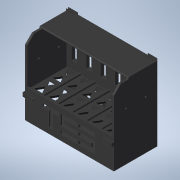
# Autodesk Inventor part: controllbox_1_copy
Saved by Autodesk Inventor 2020 (Build 240168000, 168)
## iProperties
Created: 2020-05-26
Part Number: controllbox_1_copy
Material: Generic
Document SubType Name: Modeling
Designer: Gebruiker
Density: 1 g/cm^3
Appearance: Default
Author: Gebruiker
Autodesk Inventor part; units mm, degrees
ref_plane "YZ Plane" through (0, 0, 0) normal (1, 0, 0) x (0, 1, 0)
ref_plane "XZ Plane" through (0, 0, 0) normal (0, 1, 0) x (-1, 0, 0)
ref_plane "XY Plane" through (0, 0, 0) normal (0, 0, 1) x (1, 0, 0)
sketch "Sketch1" plane through (0, 0, 0) normal (0, 0, 1) x (1, 0, 0)
  line L0 (-122.5, 65) -> (122.5, 65)
  line L1 (122.5, 65) -> (122.5, -65)
  line L2 (122.5, -65) -> (-122.5, -65)
  line L3 (-122.5, -65) -> (-122.5, 65)
  line L4 (-122.5, 65) -> (122.5, -65) construction
  line L5 (122.5, 65) -> (-122.5, -65) construction
  line L6 (-109, -65) -> (-109, 65) construction
  line L7 (-122.5, -56) -> (122.5, -56) construction
  circle A0 centre (-109, -56) radius 2
  circle A1 centre (-109, 42) radius 2
  line L8 (-109, 42) -> (122.5, 42) construction
  circle A2 centre (-69, -56) radius 2
  circle A3 centre (-29, -56) radius 2
  circle A4 centre (11, -56) radius 2
  circle A5 centre (51, -56) radius 2
  circle A6 centre (91, -56) radius 2
  line L9 (0, 65) -> (0, -65) construction
  circle A7 centre (-69, 42) radius 2
  circle A8 centre (-29, 42) radius 2
  circle A9 centre (11, 42) radius 2
  circle A10 centre (51, 42) radius 2
  circle A11 centre (91, 42) radius 2
  line L10 (-29, 42) -> (-29, -56) construction
  line L11 (-97, 65) -> (-97, -65) construction
  line L12 (-122.5, -1) -> (122.5, -1) construction
  line L13 (-104.5, 36.5) -> (-89.5, 36.5)
  line L14 (-89.5, 36.5) -> (-89.5, -38.5)
  line L15 (-89.5, -38.5) -> (-104.5, -38.5)
  line L16 (-104.5, -38.5) -> (-104.5, 36.5)
  line L17 (-104.5, 36.5) -> (-89.5, -38.5) construction
  line L18 (-89.5, 36.5) -> (-104.5, -38.5) construction
  line L19 (-64.5, 36.5) -> (-49.5, 36.5)
  line L20 (-49.5, 36.5) -> (-49.5, -38.5)
  line L21 (-64.5, -38.5) -> (-64.5, 36.5)
  line L22 (-49.5, -38.5) -> (-64.5, -38.5)
  line L23 (-24.5, 36.5) -> (-9.5, 36.5)
  line L24 (-9.5, 36.5) -> (-9.5, -38.5)
  line L25 (-24.5, -38.5) -> (-24.5, 36.5)
  line L26 (-9.5, -38.5) -> (-24.5, -38.5)
  line L27 (15.5, 36.5) -> (30.5, 36.5)
  line L28 (30.5, 36.5) -> (30.5, -38.5)
  line L29 (15.5, -38.5) -> (15.5, 36.5)
  line L30 (30.5, -38.5) -> (15.5, -38.5)
  line L31 (55.5, 36.5) -> (70.5, 36.5)
  line L32 (70.5, 36.5) -> (70.5, -38.5)
  line L33 (55.5, -38.5) -> (55.5, 36.5)
  line L34 (70.5, -38.5) -> (55.5, -38.5)
  line L35 (95.5, 36.5) -> (110.5, 36.5)
  line L36 (110.5, 36.5) -> (110.5, -38.5)
  line L37 (95.5, -38.5) -> (95.5, 36.5)
  line L38 (110.5, -38.5) -> (95.5, -38.5)
  line L39 (-105, 60.0133) -> (105, 60.0133)
  line L40 (105, 60.0133) -> (105, 50.0133)
  line L41 (105, 50.0133) -> (-105, 50.0133)
  line L42 (-105, 50.0133) -> (-105, 60.0133)
  line L43 (-105, 60.0133) -> (105, 50.0133) construction
  line L44 (105, 60.0133) -> (-105, 50.0133) construction
  point P0 (0, 0)
  point P1 (-97, -1)
  point P2 (0, 55.0133)
  dimension "d0" = 245
  dimension "d1" = 130
  dimension "d20" = 13.5
  dimension "d21" = 9
  dimension "d22" = 4
  dimension "d23" = 4
  dimension "d24" = 98
  dimension "d27" = 40
  dimension "d32" = 31.5
  dimension "d35" = 40
  dimension "d43" = 12
  dimension "d44" = 43
  dimension "d45" = 15
  dimension "d46" = 75
  dimension "d49" = 40
  dimension "d56" = 210
  dimension "d57" = 10
  dimension "d61" = 9
  constraints: 90 end point, 15 point on line, 12 centre point, 8 midpoint, 8 perpendicular, 6 horizontal, 6 parallel, 60 other
  measures "d0" distance of L1.end L2.end
  measures "d1" distance of L0.end L1.end
  measures "d20" distance between parallel lines of L6 L3
  measures "d21" distance between parallel lines of L7 L2
  measures "d22" diameter of A0
  measures "d23" diameter of A1
  measures "d24" distance of A0.centre L8.start
  measures "d27" distance of A0.centre A2.centre
  measures "d32" distance from line of L1 A6.centre
  measures "d35" distance of L8.start A7.centre
  measures "d43" distance from line of L11 L8.start
  measures "d44" distance from line of L12 L8.start
  measures "d45" distance of L14.end L15.end
  measures "d46" distance of L13.end L14.end
  measures "d49" distance of L13.start L19.start
  measures "d56" distance of L40.end L41.end
  measures "d57" distance of L39.end L40.end
  measures "d61" distance of L6.start A0.centre
extrude "Extrusion1" add sketch "Sketch1" against normal blind 10 contours L0 L1 L2 L3 | A0 | A1 | A2 | A3 | A4 | A5 | A6 | A7 | A8 | A9 | A10 | A11 | L13 L14 L15 L16 | L19 L20 L22 L21 | L23 L24 L26 L25 | L27 L28 L30 L29 | L31 L32 L34 L33 | L35 L36 L38 L37 | L39 L40 L41 L42
sketch "Sketch2" plane through (122.5, -65, 0) normal (1, 0, 0) x (0, 0, -1)
  line L0 (0, 0) -> (0, 130) projected
  line L1 (0, 0) -> (-110, 0)
  line L2 (-110, 0) -> (-110, 10)
  line L3 (-110, 10) -> (0, 10)
  line L4 (0, 10) -> (0, 0)
  point P0 (0, 65)
  dimension "d4" = 110
  dimension "d5" = 10
  constraints: 8 end point, 2 parallel, 1 horizontal, 1 perpendicular
  measures "d4" distance of L2.end L3.end
  measures "d5" distance of L1.end L2.end
extrude "Extrusion2" add sketch "Sketch2" against normal blind 245
sketch "Sketch3" plane through (122.5, -55, 110) normal (0, 1, 0) x (1, 0, 0)
  line L0 (0, 110) -> (-245, 110) projected
  line L1 (-240, 110) -> (-205, 110)
  line L2 (-205, 110) -> (-205, 5)
  line L3 (-205, 5) -> (-240, 5)
  line L4 (-240, 5) -> (-240, 110)
  line L5 (-245, 0) -> (-245, 110) projected
  line L6 (-245, 120) -> (-245, 0) projected
  line L7 (-245, 60) -> (0, 60) construction
  line L8 (0, 0) -> (0, 120) projected
  line L9 (-200, 110) -> (-165, 110)
  line L10 (-165, 110) -> (-165, 5)
  line L11 (-165, 5) -> (-200, 5)
  line L12 (-200, 5) -> (-200, 110)
  line L13 (-160, 110) -> (-125, 110)
  line L14 (-125, 110) -> (-125, 5)
  line L15 (-125, 5) -> (-160, 5)
  line L16 (-160, 5) -> (-160, 110)
  line L17 (-122.5, 110) -> (-122.5, 0) construction
  line L18 (0, 0) -> (-245, 0) construction
  line L19 (-40, 110) -> (-40, 5)
  line L20 (-40, 5) -> (-5, 5)
  line L21 (-5, 5) -> (-5, 110)
  line L22 (-80, 110) -> (-80, 5)
  line L23 (-80, 5) -> (-45, 5)
  line L24 (-45, 5) -> (-45, 110)
  line L25 (-120, 110) -> (-120, 5)
  line L26 (-120, 5) -> (-85, 5)
  line L27 (-85, 5) -> (-85, 110)
  line L28 (-234.4661, 12.7611) -> (-210.5339, 12.7611)
  line L29 (-210.5339, 12.7611) -> (-222.5, 33.6484)
  line L30 (-222.5, 33.6484) -> (-234.4661, 12.7611)
  line L31 (-222.5, 37.4721) -> (-234.4661, 56.2033)
  line L32 (-234.4661, 56.2033) -> (-210.5339, 56.2033)
  line L33 (-210.5339, 56.2033) -> (-222.5, 37.4721)
  line L34 (-210.5339, 107.2389) -> (-222.5, 86.3516)
  line L35 (-222.5, 86.3516) -> (-234.4661, 107.2389)
  line L36 (-222.5, 82.5279) -> (-234.4661, 63.7967)
  line L37 (-234.4661, 63.7967) -> (-210.5339, 63.7967)
  line L38 (-210.5339, 63.7967) -> (-222.5, 82.5279)
  line L39 (-234.4661, 107.2389) -> (-210.5339, 107.2389)
  line L40 (-205, 110) -> (-200, 110) construction
  line L41 (-200, 110) -> (-200, 5) construction
  line L42 (-200, 5) -> (-205, 5) construction
  line L43 (-205, 5) -> (-205, 110) construction
  line L44 (-202.5, 110) -> (-202.5, 5) construction
  line L45 (-170.5339, 12.7611) -> (-194.4661, 12.7611)
  line L46 (-194.4661, 12.7611) -> (-182.5, 33.6484)
  line L47 (-182.5, 33.6484) -> (-170.5339, 12.7611)
  line L48 (-182.5, 37.4721) -> (-170.5339, 56.2033)
  line L49 (-170.5339, 56.2033) -> (-194.4661, 56.2033)
  line L50 (-194.4661, 56.2033) -> (-182.5, 37.4721)
  line L51 (-194.4661, 63.7967) -> (-182.5, 82.5279)
  line L52 (-170.5339, 63.7967) -> (-194.4661, 63.7967)
  line L53 (-182.5, 82.5279) -> (-170.5339, 63.7967)
  line L54 (-182.5, 86.3516) -> (-170.5339, 107.2389)
  line L55 (-194.4661, 107.2389) -> (-182.5, 86.3516)
  line L56 (-170.5339, 107.2389) -> (-194.4661, 107.2389)
  line L57 (-165, 110) -> (-160, 110) construction
  line L58 (-160, 110) -> (-160, 5) construction
  line L59 (-160, 5) -> (-165, 5) construction
  line L60 (-165, 5) -> (-165, 110) construction
  line L61 (-162.5, 110) -> (-162.5, 5) construction
  line L62 (-130.5339, 12.7611) -> (-142.5, 33.6484)
  line L63 (-142.5, 33.6484) -> (-154.4661, 12.7611)
  line L64 (-154.4661, 12.7611) -> (-130.5339, 12.7611)
  line L65 (-142.5, 37.4721) -> (-154.4661, 56.2033)
  line L66 (-130.5339, 56.2033) -> (-142.5, 37.4721)
  line L67 (-154.4661, 56.2033) -> (-130.5339, 56.2033)
  line L68 (-154.4661, 63.7967) -> (-130.5339, 63.7967)
  line L69 (-130.5339, 63.7967) -> (-142.5, 82.5279)
  line L70 (-142.5, 82.5279) -> (-154.4661, 63.7967)
  line L71 (-142.5, 86.3516) -> (-154.4661, 107.2389)
  line L72 (-130.5339, 107.2389) -> (-142.5, 86.3516)
  line L73 (-154.4661, 107.2389) -> (-130.5339, 107.2389)
  line L74 (-10.5339, 12.7611) -> (-34.4661, 12.7611)
  line L75 (-22.5, 33.6484) -> (-10.5339, 12.7611)
  line L76 (-22.5, 37.4721) -> (-10.5339, 56.2033)
  line L77 (-10.5339, 56.2033) -> (-34.4661, 56.2033)
  line L78 (-34.4661, 56.2033) -> (-22.5, 37.4721)
  line L79 (-34.4661, 63.7967) -> (-22.5, 82.5279)
  line L80 (-10.5339, 63.7967) -> (-34.4661, 63.7967)
  line L81 (-22.5, 82.5279) -> (-10.5339, 63.7967)
  line L82 (-22.5, 86.3516) -> (-10.5339, 107.2389)
  line L83 (-34.4661, 107.2389) -> (-22.5, 86.3516)
  line L84 (-10.5339, 107.2389) -> (-34.4661, 107.2389)
  line L85 (-50.5339, 12.7611) -> (-62.5, 33.6484)
  line L86 (-74.4661, 12.7611) -> (-50.5339, 12.7611)
  line L87 (-62.5, 37.4721) -> (-74.4661, 56.2033)
  line L88 (-50.5339, 56.2033) -> (-62.5, 37.4721)
  line L89 (-74.4661, 56.2033) -> (-50.5339, 56.2033)
  line L90 (-74.4661, 63.7967) -> (-50.5339, 63.7967)
  line L91 (-50.5339, 63.7967) -> (-62.5, 82.5279)
  line L92 (-62.5, 82.5279) -> (-74.4661, 63.7967)
  line L93 (-62.5, 86.3516) -> (-74.4661, 107.2389)
  line L94 (-50.5339, 107.2389) -> (-62.5, 86.3516)
  line L95 (-74.4661, 107.2389) -> (-50.5339, 107.2389)
  line L96 (-102.5, 33.6484) -> (-90.5339, 12.7611)
  line L97 (-90.5339, 12.7611) -> (-114.4661, 12.7611)
  line L98 (-114.4661, 12.7611) -> (-102.5, 33.6484)
  line L99 (-114.4661, 56.2033) -> (-102.5, 37.4721)
  line L100 (-102.5, 37.4721) -> (-90.5339, 56.2033)
  line L101 (-90.5339, 56.2033) -> (-114.4661, 56.2033)
  line L102 (-90.5339, 63.7967) -> (-114.4661, 63.7967)
  line L103 (-102.5, 82.5279) -> (-90.5339, 63.7967)
  line L104 (-114.4661, 63.7967) -> (-102.5, 82.5279)
  line L105 (-114.4661, 107.2389) -> (-102.5, 86.3516)
  line L106 (-102.5, 86.3516) -> (-90.5339, 107.2389)
  line L107 (-90.5339, 107.2389) -> (-114.4661, 107.2389)
  line L108 (-74.4661, 12.7611) -> (-62.5, 33.6484)
  line L109 (-34.4661, 12.7611) -> (-22.5, 33.6484)
  dimension "d8" = 35
  dimension "d9" = 105
  dimension "d10" = 5
  dimension "d11" = 35
  dimension "d12" = 35
  dimension "d13" = 105
  dimension "d14" = 5
  dimension "d15" = 5
  constraints: 210 end point, 78 symmetric about line, 10 parallel, 8 horizontal, 7 midpoint, 5 perpendicular, 3 equal length, 3 point on line
  measures "d8" distance of L2.end L3.end
  measures "d9" distance of L1.end L2.end
  measures "d10" distance between parallel lines of L4 L5
  measures "d11" distance of L10.end L11.end
  measures "d12" distance of L14.end L15.end
  measures "d13" distance of L13.end L14.end
  measures "d14" distance between parallel lines of L12 L2
  measures "d15" distance between parallel lines of L16 L10
extrude "Extrusion3" cut sketch "Sketch3" against normal blind 5 contours L21 L20 L19 L0 | L2 L3 L4 L0 | L10 L11 L12 L0 | L14 L15 L16 L0 | L27 L26 L25 L0 | L24 L23 L22 L0 | L30 L29 L28 | L31 L32 L33 | L34 L35 L39 | L38 L37 L36 | L45 L46 L47 | L50 L49 L48 | L51 L53 L52 | L55 L56 L54 | L64 L63 L62 | L65 L67 L66 | L70 L69 L68 | L71 L73 L72 | L74 L109 L75 | L78 L77 L76 | L79 L81 L80 | L83 L84 L82 | L86 L108 L85 | L87 L89 L88 | L92 L91 L90 | L93 L95 L94 | L96 L97 L98 | L101 L100 L99 | L102 L104 L103 | L107 L106 L105
extrude "Extrusion4" cut sketch "Sketch3" against normal blind 10 contours L30 L29 L28 | L31 L32 L33 | L34 L35 L39 | L38 L37 L36 | L45 L46 L47 | L50 L49 L48 | L51 L53 L52 | L55 L56 L54 | L64 L63 L62 | L65 L67 L66 | L70 L69 L68 | L71 L73 L72 | L74 L109 L75 | L78 L77 L76 | L79 L81 L80 | L83 L84 L82 | L86 L108 L85 | L87 L89 L88 | L92 L91 L90 | L93 L95 L94 | L96 L97 L98 | L101 L100 L99 | L102 L104 L103 | L107 L106 L105
extrude "Extrusion5" cut sketch "Sketch1" against normal blind 10 contours A0 | A1 | A2 | A3 | A4 | A5 | A6 | A7 | A8 | A9 | A10 | A11
extrude "Extrusion6" cut sketch "Sketch1" against normal blind 10 contours L13 L14 L15 L16 | L19 L20 L22 L21 | L23 L24 L26 L25 | L27 L28 L30 L29 | L31 L32 L34 L33 | L35 L36 L38 L37
extrude "Extrusion7" cut sketch "Sketch1" against normal blind 10 contours L39 L40 L41 L42
fillet "Fillet1" radius 2 4 edges at (-105, 50.0133, -5) (-105, 60.0133, -5) (105, 50.0133, -5) (105, 60.0133, -5)
sketch "Sketch4" plane through (122.5, -65, 110) normal (0, 0, 1) x (1, 0, 0)
  line L0 (0, 10) -> (-245, 10) projected
  line L1 (-245, 10) -> (-240, 10)
  line L2 (-240, 10) -> (-240, 130)
  line L3 (-240, 130) -> (-245, 130)
  line L4 (-245, 130) -> (-245, 10)
  line L5 (0, 130) -> (-245, 130) projected
  line L6 (0, 10) -> (-5, 10)
  line L7 (-5, 10) -> (-5, 130)
  line L8 (-5, 130) -> (0, 130)
  line L9 (0, 130) -> (0, 10)
  line L10 (0, 120) -> (0, 125)
  point P0 (-122.5, 65)
  point P1 (-245, 125)
  dimension "d62" = 5
  dimension "d63" = 120
  dimension "d64" = 0
  dimension "d66" = 120
  dimension "d69" = 5
  constraints: 18 end point, 4 parallel, 2 horizontal, 2 perpendicular
  measures "d62" distance of L3.end L2.end
  measures "d63" distance of L2.end L1.end
  measures "d64" distance between parallel lines of L5 L3
  measures "d66" distance of L6.end L7.end
  measures "d69" distance of L10.end L10.start
extrude "Extrusion8" add sketch "Sketch4" against normal blind 110 contours L0 L7 L5 L9 | L0 L4 L3 L2
sketch "Sketch5" plane through (122.5, -65, -10) normal (1, 0, 0) x (0, 0, -1)
  line L0 (0, 0) -> (0, 130) projected
  line L1 (0, 130) -> (-80, 130)
  line L2 (-80, 130) -> (-80, 135)
  line L3 (-80, 135) -> (0, 135)
  line L4 (0, 135) -> (0, 130)
  point P0 (-10, 65)
  dimension "d70" = 80
  dimension "d71" = 5
  constraints: 8 end point, 2 parallel, 1 horizontal, 1 perpendicular
  measures "d70" distance of L2.end L3.end
  measures "d71" distance of L1.end L2.end
extrude "Extrusion9" add sketch "Sketch5" against normal blind 245
fillet "Fillet2" radius 2 4 edges at (120, 65, 70) (0, 70, 70) (-120, 65, 70) (0, 65, 70)
sketch "Sketch11" plane through (-122.5, -65, -10) normal (0, -1, 0) x (1, 0, 0)
  line L0 (0, 0) -> (0, 120) projected
  line L1 (245, 120) -> (245, 0) projected
  line L2 (0, 0) -> (245, 0)
  line L3 (245, 0) -> (245, 5)
  line L4 (245, 5) -> (0, 5)
  line L5 (0, 5) -> (0, 0)
  line L6 (240, 120) -> (240, 115) projected
  line L7 (245, 0) -> (240, 0)
  line L8 (240, 0) -> (240, 120)
  line L9 (240, 120) -> (245, 120)
  line L10 (245, 120) -> (245, 0)
  line L11 (245, 120) -> (0, 120) projected
  line L12 (245, 120) -> (0, 120)
  line L13 (0, 120) -> (0, 115)
  line L14 (0, 115) -> (245, 115)
  line L15 (245, 115) -> (245, 120)
  point P0 (122.5, 10)
  point P1 (240, 5)
  dimension "d103" = 5
  constraints: 24 end point, 6 parallel, 3 horizontal, 3 perpendicular, 2 point on line
  measures "d103" distance of L3.end L2.end
extrude "Extrusion13" add sketch "Sketch11" along normal blind 65 contours L0 L4 L8 L2 | L8 L4 L1 L2 | L0 L11 L6 L14 | L8 L14 L1 L4 | L6 L9 L1 L14
sketch "Sketch12" plane through (122.5, 70, 68) normal (1, 0, 0) x (0, 0, -1)
  line L0 (78, -200) -> (-42, -200) projected
  line L1 (78, -200) -> (-42, -200)
  line L2 (-42, -200) -> (-42, -205)
  line L3 (-42, -205) -> (78, -205)
  line L4 (78, -205) -> (78, -200)
  point P0 (68, -70)
  dimension "d106" = 5
  constraints: 8 end point, 2 parallel, 1 horizontal, 1 perpendicular
  measures "d106" distance of L2.end L1.end
extrude "Extrusion14" add sketch "Sketch12" against normal blind 245
sketch "Sketch13" plane through (117.5, -55, 110) normal (0, 0, 1) x (1, 0, 0)
  line L0 (-240, 125) -> (-240, -80) construction
  line L1 (5, 120) -> (5, -80) construction
  line L2 (5, -80) -> (-240, -80) construction
  line L3 (5, -0.0002) -> (-240, -80) construction
  line L4 (-240, -40.0001) -> (5, -40.0001) construction
  line L5 (-192.5, -15.0001) -> (-42.5, -15.0001)
  line L6 (-42.5, -15.0001) -> (-42.5, -65.0001)
  line L7 (-42.5, -65.0001) -> (-192.5, -65.0001)
  line L8 (-192.5, -65.0001) -> (-192.5, -15.0001)
  line L9 (-42.5, -15.0001) -> (-192.5, -65.0001) construction
  line L10 (-192.5, -15.0001) -> (-147.5, -15.0001)
  line L11 (-147.5, -15.0001) -> (-147.5, -25.0001)
  line L12 (-147.5, -25.0001) -> (-192.5, -25.0001)
  line L13 (-192.5, -25.0001) -> (-192.5, -15.0001)
  line L14 (-175, -15.0001) -> (-165, -15.0001)
  line L15 (-165, -15.0001) -> (-165, -65.0001)
  line L16 (-165, -65.0001) -> (-175, -65.0001)
  line L17 (-175, -65.0001) -> (-175, -15.0001)
  line L18 (-175, -15.0001) -> (-165, -65.0001) construction
  line L19 (-165, -15.0001) -> (-175, -65.0001) construction
  line L20 (-97.5, -15.0001) -> (-142.5, -15.0001)
  line L21 (-142.5, -15.0001) -> (-142.5, -25.0001)
  line L22 (-142.5, -25.0001) -> (-97.5, -25.0001)
  line L23 (-97.5, -25.0001) -> (-97.5, -15.0001)
  line L24 (-47.5, -15.0001) -> (-92.5, -15.0001)
  line L25 (-92.5, -15.0001) -> (-92.5, -25.0001)
  line L26 (-92.5, -25.0001) -> (-47.5, -25.0001)
  line L27 (-47.5, -25.0001) -> (-47.5, -15.0001) construction
  line L28 (-142.5, -35.0001) -> (-97.5, -35.0001)
  line L29 (-97.5, -35.0001) -> (-97.5, -45.0001)
  line L30 (-97.5, -45.0001) -> (-142.5, -45.0001)
  line L31 (-142.5, -45.0001) -> (-142.5, -35.0001)
  line L32 (-142.5, -35.0001) -> (-97.5, -45.0001) construction
  line L33 (-97.5, -35.0001) -> (-142.5, -45.0001) construction
  line L34 (-92.5, -34.634) -> (-47.5, -34.634)
  line L35 (-47.5, -34.634) -> (-47.5, -45.0001)
  line L36 (-47.5, -45.0001) -> (-92.5, -45.0001)
  line L37 (-92.5, -45.0001) -> (-92.5, -34.634)
  line L38 (-92.5, -34.634) -> (-47.5, -45.0001) construction
  line L39 (-47.5, -34.634) -> (-92.5, -45.0001) construction
  line L40 (-97.5, -65.0001) -> (-142.5, -65.0001)
  line L41 (-142.5, -65.0001) -> (-142.5, -55.0001)
  line L42 (-142.5, -55.0001) -> (-97.5, -55.0001)
  line L43 (-97.5, -55.0001) -> (-97.5, -65.0001)
  line L44 (-47.5, -65.0001) -> (-92.5, -65.0001)
  line L45 (-92.5, -65.0001) -> (-92.5, -55.0001)
  line L46 (-92.5, -55.0001) -> (-47.5, -55.0001)
  line L47 (-47.5, -55.0001) -> (-47.5, -65.0001)
  line L48 (-47.5, -25.0001) -> (-47.5, -15.0001)
  line L49 (-47.5, -45.0001) -> (-47.5, -55.0001) construction
  line L50 (-142.5, -25.0001) -> (-132.5, -25.0001)
  line L51 (-132.5, -25.0001) -> (-132.5, -35.0001)
  line L52 (-132.5, -35.0001) -> (-142.5, -35.0001)
  line L53 (-142.5, -35.0001) -> (-142.5, -25.0001)
  line L54 (-47.5, -45.0001) -> (-57.5, -45.0001)
  line L55 (-57.5, -45.0001) -> (-57.5, -55.0001)
  line L56 (-57.5, -55.0001) -> (-47.5, -55.0001)
  line L57 (-47.5, -55.0001) -> (-47.5, -45.0001)
  point P0 (-117.5, 55)
  point P1 (-117.5, -40.0001)
  point P2 (-170, -40.0001)
  point P3 (-120, -40.0001)
  point P4 (-70, -39.817)
  point P5 (-92.5, -65.0001)
  point P6 (-142.5, -15.0001)
  point P7 (-175, -25.0001)
  point P8 (-175, -65.0001)
  point P9 (-165, -25.0001)
  point P10 (-192.5, -25.0001)
  point P11 (-92.5, -15.0001)
  point P12 (-47.5, -55.0001)
  point P13 (-57.5, -45.0001)
  point P14 (-142.5, -35.0001)
  point P15 (-132.5, -25.0001)
  dimension "d109" = 150
  dimension "d110" = 50
  dimension "d111" = 45
  dimension "d112" = 10
  dimension "d113" = 10
  dimension "d116" = 45
  dimension "d117" = 10
  dimension "d118" = 5
  dimension "d119" = 45
  dimension "d120" = 10
  dimension "d121" = 45
  dimension "d122" = 10
  dimension "d123" = 10
  dimension "d132" = 10
  dimension "d133" = 10
  dimension "d134" = 10
  dimension "d135" = 10
  constraints: 110 end point, 22 parallel, 12 horizontal, 12 perpendicular, 12 point on line, 8 midpoint, 1 vertical
  measures "d109" distance of L6.end L7.end
  measures "d110" distance of L5.end L6.end
  measures "d111" distance of L11.end L12.end
  measures "d112" distance of L10.end L11.end
  measures "d113" distance of L15.end L16.end
  measures "d116" distance of L26.end L25.end
  measures "d117" distance of L25.end L24.end
  measures "d118" distance between parallel lines of L25 L23
  measures "d119" distance of L29.end L30.end
  measures "d120" distance of L28.end L29.end
  measures "d121" distance of L35.end L36.end
  measures "d122" distance of L40.end L41.end
  measures "d123" distance of L44.end L45.end
  measures "d132" distance between parallel lines of L28 L22
  measures "d133" distance between parallel lines of L42 L30
  measures "d134" distance of L51.end L52.end
  measures "d135" distance of L56.end L55.end
extrude "Extrusion15" cut sketch "Sketch13" against normal blind 5 contours L5 L17 L12 L8 | L5 L15 L12 L17 | L5 L11 L12 L15 | L12 L15 L7 L17 | L5 L23 L22 L21 | L22 L51 L28 L53 | L41 L42 L43 L7 | L5 L48 L26 L25 | L28 L29 L30 L31 | L45 L46 L47 L7 | L46 L55 L36 L57 | L36 L37 L34 L35
sketch "Sketch14" plane through (0, 0, -10) normal (0, 0, -1) x (-1, 0, 0)
  line L0 (-73.9071, -63.6856) -> (76.0929, -63.6856)
  line L1 (76.0929, -63.6856) -> (76.0929, -113.6856)
  line L2 (76.0929, -113.6856) -> (-73.9071, -113.6856)
  line L3 (-73.9071, -113.6856) -> (-73.9071, -63.6856)
  line L4 (-73.9071, -63.6856) -> (-28.9071, -63.6856)
  line L5 (-28.9071, -63.6856) -> (-28.9071, -73.6856)
  line L6 (-28.9071, -73.6856) -> (-73.9071, -73.6856)
  line L7 (-73.9071, -73.6856) -> (-73.9071, -63.6856)
  line L8 (-56.4071, -63.6856) -> (-46.4071, -63.6856)
  line L9 (-46.4071, -63.6856) -> (-46.4071, -113.6856)
  line L10 (-46.4071, -113.6856) -> (-56.4071, -113.6856)
  line L11 (-56.4071, -113.6856) -> (-56.4071, -63.6856)
  line L12 (21.0929, -63.6856) -> (-23.9071, -63.6856)
  line L13 (-23.9071, -63.6856) -> (-23.9071, -73.6856)
  line L14 (-23.9071, -73.6856) -> (21.0929, -73.6856)
  line L15 (21.0929, -73.6856) -> (21.0929, -63.6856)
  line L16 (71.0929, -63.6856) -> (26.0929, -63.6856)
  line L17 (26.0929, -63.6856) -> (26.0929, -73.6856)
  line L18 (26.0929, -73.6856) -> (71.0929, -73.6856)
  line L19 (71.0929, -73.6856) -> (71.0929, -63.6856) construction
  line L20 (-23.9071, -83.6856) -> (21.0929, -83.6856)
  line L21 (21.0929, -83.6856) -> (21.0929, -93.6856)
  line L22 (21.0929, -93.6856) -> (-23.9071, -93.6856)
  line L23 (-23.9071, -93.6856) -> (-23.9071, -83.6856)
  line L24 (26.0929, -83.3195) -> (71.0929, -83.3195)
  line L25 (71.0929, -83.3195) -> (71.0929, -93.6856)
  line L26 (71.0929, -93.6856) -> (26.0929, -93.6856)
  line L27 (26.0929, -93.6856) -> (26.0929, -83.3195)
  line L28 (21.0929, -113.6856) -> (-23.9071, -113.6856)
  line L29 (-23.9071, -113.6856) -> (-23.9071, -103.6856)
  line L30 (-23.9071, -103.6856) -> (21.0929, -103.6856)
  line L31 (21.0929, -103.6856) -> (21.0929, -113.6856)
  line L32 (71.0929, -113.6856) -> (26.0929, -113.6856)
  line L33 (26.0929, -113.6856) -> (26.0929, -103.6856)
  line L34 (26.0929, -103.6856) -> (71.0929, -103.6856)
  line L35 (71.0929, -103.6856) -> (71.0929, -113.6856)
  line L36 (71.0929, -73.6856) -> (71.0929, -63.6856)
  line L37 (71.0929, -93.6856) -> (71.0929, -103.6856) construction
  line L38 (-23.9071, -73.6856) -> (-13.9071, -73.6856)
  line L39 (-13.9071, -73.6856) -> (-13.9071, -83.6856)
  line L40 (-13.9071, -83.6856) -> (-23.9071, -83.6856)
  line L41 (-23.9071, -83.6856) -> (-23.9071, -73.6856)
  line L42 (71.0929, -93.6856) -> (61.0929, -93.6856)
  line L43 (61.0929, -93.6856) -> (61.0929, -103.6856)
  line L44 (61.0929, -103.6856) -> (71.0929, -103.6856)
  line L45 (71.0929, -103.6856) -> (71.0929, -93.6856)
  line L46 (-122.5, -135) -> (-122.5, 70) projected
  line L47 (122.5, 70) -> (122.5, -135) projected
  point P0 (0, 0)
  point P1 (-56.4071, -73.6856)
  point P2 (-46.4071, -73.6856)
  dimension "d136" = 150
  dimension "d137" = 50
  dimension "d138" = 45
  dimension "d139" = 10
  dimension "d140" = 10
  dimension "d141" = 45
  dimension "d142" = 10
  dimension "d143" = 5
  dimension "d144" = 45
  dimension "d145" = 10
  dimension "d146" = 45
  dimension "d147" = 10
  dimension "d148" = 10
  dimension "d149" = 10
  dimension "d150" = 10
  dimension "d151" = 10
  dimension "d152" = 10
  dimension "d154" = 46.4071
  constraints: 92 end point, 22 parallel, 12 perpendicular, 11 horizontal, 8 point on line, 1 vertical
  measures "d136" distance of L2.start L3.start
  measures "d137" distance of L0.end L2.start
  measures "d138" distance of L5.end L6.end
  measures "d139" distance of L5.start L5.end
  measures "d140" distance of L9.end L10.end
  measures "d141" distance of L19.start L18.start
  measures "d142" distance of L18.start L16.end
  measures "d143" distance between parallel lines of L17 L15
  measures "d144" distance of L21.end L23.start
  measures "d145" distance of L20.end L21.end
  measures "d146" distance of L42.start L26.end
  measures "d147" distance of L29.start L29.end
  measures "d148" distance of L32.end L34.start
  measures "d149" distance between parallel lines of L20 L14
  measures "d150" distance between parallel lines of L30 L22
  measures "d151" distance of L39.end L40.end
  measures "d152" distance of L45.start L43.end
  measures "d154" distance between parallel lines of L47 L1
extrude "Extrusion16" cut sketch "Sketch14" against normal blind 5 contours L0 L11 L6 L3 | L0 L9 L6 L11 | L0 L5 L6 L9 | L6 L9 L2 L11 | L0 L15 L14 L13 | L14 L39 L20 L41 | L29 L30 L31 L2 | L0 L36 L18 L17 | L20 L21 L22 L23 | L33 L34 L35 L2 | L34 L43 L26 L45 | L26 L27 L24 L25
sketch "Sketch15" plane through (117.5, -55, 110) normal (0, 0, 1) x (1, 0, 0)
  line L0 (-240, -10) -> (5, -10)
  line L1 (-240, -10) -> (-215, -10) construction
  line L2 (-215, -10) -> (-215, -20)
  line L3 (-215, -20) -> (-240, -20)
  line L4 (-240, -20) -> (-240, -10) construction
  line L5 (-240, -10) -> (-240, -20) construction
  line L6 (-240, -10) -> (-188.5929, -10) construction
  line L7 (-240, -10) -> (-215, -10) construction
  line L8 (-240, -10) -> (-240, -20)
  line L9 (5, -10) -> (-20, -10)
  line L10 (-20, -10) -> (-20, -20)
  line L11 (-20, -20) -> (5, -20)
  line L12 (5, -20) -> (5, -10)
  point P0 (-117.5, 55)
  point P1 (-20, -10)
  dimension "d158" = 245
  dimension "d159" = 25
  dimension "d160" = 10
  dimension "d161" = 25
  dimension "d162" = 10
  constraints: 24 end point, 4 parallel, 3 horizontal, 2 perpendicular, 1 collinear, 1 vertical
  measures "d158" distance of L0.start L0.end
  measures "d159" distance of L2.end L3.end
  measures "d160" distance of L1.end L2.end
  measures "d161" distance of L11.end L10.end
  measures "d162" distance of L10.end L9.end
extrude "Extrusion17" add sketch "Sketch15" along normal blind 7
sketch "Sketch16" plane through (-122.5, -65, 110) normal (0, 1, 0) x (1, 0, 0)
  line L0 (47.5, -6) -> (2.5, -6)
  line L1 (2.5, -6) -> (2.5, -1)
  line L2 (2.5, -1) -> (47.5, -1)
  line L3 (47.5, -1) -> (47.5, -6)
  line L4 (25, 0) -> (25, -7) projected
  line L5 (47.5, -6) -> (2.5, -1) construction
  line L6 (2.5, -6) -> (47.5, -1) construction
  line L7 (197.5, -1) -> (242.5, -1)
  line L8 (242.5, -1) -> (242.5, -6)
  line L9 (242.5, -6) -> (197.5, -6)
  line L10 (197.5, -6) -> (197.5, -1)
  line L11 (220, 0) -> (220, -7) projected
  line L12 (197.5, -1) -> (242.5, -6) construction
  line L13 (242.5, -1) -> (197.5, -6) construction
  point P0 (122.5, 110)
  point P1 (25, -3.5)
  point P2 (220, -3.5)
  point P3 (220, -1)
  point P4 (220, -6)
  point P5 (25, -6)
  point P6 (25, -1)
  dimension "d165" = 45
  dimension "d166" = 5
  dimension "d167" = 45
  dimension "d168" = 5
  constraints: 24 end point, 6 midpoint, 4 parallel, 2 horizontal, 2 perpendicular
  measures "d165" distance of L1.end L2.end
  measures "d166" distance of L0.end L1.end
  measures "d167" distance of L8.end L9.end
  measures "d168" distance of L7.end L8.end
extrude "Extrusion18" cut sketch "Sketch16" against normal blind 7 contours L0 L1 L2 L4 | L7 L8 L9 L11
sketch "Sketch18" plane through (-122.5, 70, -10) normal (0, 1, 0) x (1, 0, 0)
  line L0 (245, 0) -> (0, 0) projected
  line L1 (245, 0) -> (220, 0)
  line L2 (220, 0) -> (220, -7)
  line L3 (220, -7) -> (245, -7)
  line L4 (245, -7) -> (245, 0)
  line L5 (0, -78) -> (0, 0) projected
  line L6 (0, 0) -> (25, 0)
  line L7 (25, 0) -> (25, -7)
  line L8 (25, -7) -> (0, -7)
  line L9 (0, -7) -> (0, 0)
  line L10 (245, -6) -> (220, -6)
  line L11 (220, -6) -> (220, -1)
  line L12 (220, -1) -> (245, -1)
  line L13 (245, -1) -> (245, -6)
  line L14 (245, -6) -> (220, -1) construction
  line L15 (220, -6) -> (245, -1) construction
  line L16 (25, -6) -> (0, -6)
  line L17 (0, -6) -> (0, -1)
  line L18 (0, -1) -> (25, -1)
  line L19 (25, -1) -> (25, -6)
  line L20 (25, -6) -> (0, -1) construction
  line L21 (0, -6) -> (25, -1) construction
  point P0 (122.5, -10)
  point P1 (232.5, -3.5)
  point P2 (12.5, -3.5)
  point P3 (245, -1)
  point P4 (220, 0)
  point P5 (0, -1)
  point P6 (25, -1)
  point P7 (25, -6)
  point P8 (0, -6)
  point P9 (0, -7)
  dimension "d177" = 25
  dimension "d178" = 7
  dimension "d179" = 25
  dimension "d180" = 7
  dimension "d181" = 5
  dimension "d182" = 5
  constraints: 40 end point, 8 parallel, 4 horizontal, 4 midpoint, 4 perpendicular, 2 point on line
  measures "d177" distance of L3.end L2.end
  measures "d178" distance of L1.end L2.end
  measures "d179" distance of L7.end L8.end
  measures "d180" distance of L6.end L7.end
  measures "d181" distance of L10.end L11.end
  measures "d182" distance of L16.end L17.end
extrude "Extrusion20" add sketch "Sketch18" along normal blind 5 contours L4 L12 L2 L0 | L7 L18 L5 L0 | L4 L3 L2 L10 | L7 L8 L5 L16
sketch "Sketch22" plane through (117.5, -55, 110) normal (-1, 0, 0) x (0, 0, 1)
  line L0 (0, 120) -> (-38, 120) projected
  line L1 (-19, 120) -> (-2.2692, 103.2692)
  line L2 (-19, 120) -> (4.661, 120) construction
  line L3 (-2.2692, 103.2692) -> (0, 101)
  line L4 (0, 120) -> (0, -10) projected
  point P0 (-110, 55)
  dimension "d188" = 45
  constraints: 6 end point, 2 point on line, 1 equal length, 1 horizontal, 1 midpoint
  measures "d188" angle of L1 L2
extrude "Extrusion22" cut sketch "Sketch22" against normal blind 5
sketch "Sketch24" plane through (-122.5, 65, 72) normal (-1, 0, 0) x (0, 0, 1)
  line L0 (38, 0) -> (0, 0) projected
  line L1 (38, -19) -> (38, -130) projected
  line L2 (19, 0) -> (38, -19)
  line L3 (38, -19) -> (38, 0)
  line L4 (38, 0) -> (19, 0)
  point P0 (-72, -65)
  constraints: 6 end point, 1 collinear, 1 midpoint, 1 perpendicular
extrude "Extrusion23" cut sketch "Sketch24" against normal blind 5
fillet "Fillet3" radius 4 2 edges at (-120, 65, 91) (120, 65, 91)
sketch "Sketch25" plane through (-122.5, -135, -10) normal (-1, 0, 0) x (0, 0, 1)
  line L0 (0, 96.5) -> (0, 171.5) construction
  line L1 (0, 134) -> (120, 134) construction
  line L2 (120, 179.3431) -> (120, 80) construction
  circle A0 centre (32.2426, 134) radius 10
  circle A1 centre (87.2426, 134) radius 10
  line L3 (22.5, 144) -> (97.5, 144)
  line L4 (97.5, 144) -> (97.5, 124)
  line L5 (97.5, 124) -> (22.5, 124)
  line L6 (22.5, 124) -> (22.5, 144)
  line L7 (22.5, 144) -> (97.5, 124) construction
  line L8 (97.5, 144) -> (22.5, 124) construction
  circle A2 centre (87.2426, 134) radius 2
  circle A3 centre (32.2426, 134) radius 2
  point P0 (10, 135)
  point P1 (60, 134)
  point P2 (32.2426, 124)
  point P3 (87.2426, 124)
  point P4 (87.2426, 144)
  point P5 (32.2426, 144)
  dimension "d195" = 20
  dimension "d196" = 20
  dimension "d197" = 55
  dimension "d200" = 75
  dimension "d213" = 4
  dimension "d214" = 4
  constraints: 14 end point, 4 centre point, 4 midpoint, 3 point on line, 2 coincident, 2 horizontal, 2 parallel, 1 perpendicular
  measures "d195" diameter of A0
  measures "d196" diameter of A1
  measures "d197" distance of A1.centre A0.centre
  measures "d200" distance of L4.end L5.end
  measures "d213" diameter of A2
  measures "d214" diameter of A3
extrude "Extrusion27" cut sketch "Sketch25" against normal blind 5 contours A2 | A3
mirror "Mirror2" about plane through (0, 0, 0) normal (1, 0, 0) of "Extrusion27"
body "Solid1"
